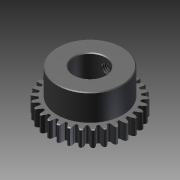
# Autodesk Inventor part: GEAB1.0-30-6-B-12_b
Saved by Autodesk Inventor 2011 SP1 (Build 150282100, 282)
## iProperties
Created: 2016-10-27
Part Number: GEAB1.0-30-6-B-12_b
Catalog Web Link: www.cadenas.de
Description: GEAHB1.0, GEAHBB1.0, GEAHBG1.0, GEAHS1.0, GEAB1.0, GEABB1.0, GEABG1.0, GEAS1.0, GEAKB1.0, GEAKBB1.0, GEAKBG1.0, GEAKS1.0_body-Spur Gears - Pressure Angle 20 Degree Module 1.0
Vendor: MISUMI
Document SubType Name: Modeling
Designer: psAdmin
Manufacturer: MISUMI
Mass: 7.21625 g
Surface Area: 36.7251 cm^2
Volume: 7.21625 cm^3
Density: 1 g/cm^3
Category: PARTsolutions
Company: MISUMI
Title: GEAB1.0-30-6-B-12
Author: Cadenas PARTsolutions
Comments: Spur Gears - Pressure Angle 20 Degree Module 1.0
PSOL_IDENT_0: {$CADENAS_DATA\23d-libs\misumi\metric\54_spur_gears\geab10\geab10.prj},462 {VTYP=3D},{NB=GEAB1.0-30-
PSOL_IDENT_1: 6-B-12_b},{LINA=GEAB1.0-30-6-B-12},{NN=GEAHB1.0, GEAHBB1.0, GEAHBG1.0, GEAHS1.0, GEAB1.0, GEABB1.0,
PSOL_IDENT_2: GEABG1.0, GEAS1.0, GEAKB1.0, GEAKBB1.0, GEAKBG1.0, GEAKS1.0_body},{DATE=13.09.2016 11:19:06},{GEOMDA
PSOL_IDENT_3: TE=13.09.2016 06:08:24},{VERSION=},{LINEID=20},{LINESUBID=-1},{WBVAR=SHS,MAT,ST,NT,B,TS,PS,ALT1,ALT2
PSOL_IDENT_4: ,TPC,ALT11,ALT10,BS,ALT4,Z,J,ALT5,Q,R,S,T,ALT9,SRG,ALT6,LFC,LTC,MALT6,ALT7,KFC,KTC,K,ALT3,DIRALT3,QF
PSOL_IDENT_5: C,QTC,MALT3,ALT8,DIRALT8,ZFC,ZTC,U}  {NB=GEAB1.0-30-6-B-12_b},{LINA=GEAB1.0-30-6-B-12},{KT=DUMMY},{P
PSOL_IDENT_6: N=GEAB1.0-30-6-B-12},{SHS=RHT},{TYPE=GEAB},{MAT=S45C},{MATALG= 'S45C','S45C Equivalent','SUS304','SU
PSOL_IDENT_7: S304' },{ST=},{STALG= '','-','BO','Black Oxide','ENP','Electroless Nickel Plating'},{AC=Set Screw(41
PSOL_IDENT_8: 37 Alloy Steel Black Oxide)},{MOD=1.0},{NT=30},{NTALG=12,13,14,15,16,17,18,19,20,21,22,23,24,25,26,2
PSOL_IDENT_9: 7,28,29,30,32,34,35,36,38,40,42,44,45,46,48,50,52,54,55,56,58,60,62,64,65,66,68,70,72,75,80,84,85,90
PSOL_IDENT_10: ,95,96,100,110,120},{B=6},{BALG=6,8,10,12},{TS=B},{TSALG='B','B'},{TSPN=-B},{PS=12},{PSALG='6','6','
PSOL_IDENT_11: 6.35','6.35','7','7','8','8','9','9','10','10','11','11','12','12','13','13','14','14','15','15','16'
PSOL_IDENT_12: ,'16','17','17'},{P=12.00},{DD=30},{D=32},{G=27.5},{H=25},{L=16},{LL1=10},{LL2=4},{M=M4},{ML=6.500},
PSOL_IDENT_13: {ALT1=},{ALT1ALG='', 'w/o Set Screw', 'KC90','with KC90 (Set Screw)','KC120','with KC120 (Set Screw)'
PSOL_IDENT_14: },{ALT1PN=},{KC=0},{ALT2=},{ALT2ALG= '','w/o TPC (Tapped Hole Dimension)','TPC','with TPC (Tapped H
PSOL_IDENT_15: ole Dimension)' },{TPC=N/A},{TPCALG= 'N/A' },{ALT2PN=},{ALT11=},{ALT11ALG= '', 'w/o GBA (Gear bottom
PSOL_IDENT_16: adjustment of phase focus)','GBA','with GBA (Gear bottom adjustment of phase focus)' },{ALT11PN=},{
PSOL_IDENT_17: DEG=0},{ALT10=},{ALT10ALG= '','w/o BS (Boss Cut)','BS','with BS (Boss Cut)' },{BS=0.0},{BSALG=0},{BS
PSOL_IDENT_18: MIN=7},{BSMAX=10},{ALT10PN=},{LL13D=10},{LL23D=12},{LBS=16},{ALT4=},{ALT4ALG= '','N/A' },{ALT41=0},{
PSOL_IDENT_19: ALT42=0},{ALT4PN=},{Z=0},{ZALG=0},{ZPN=},{ZMINL=14},{ZMAXL=23},{ZMINR=14},{ZMAXR=21},{J=0.0},{JALG=0
PSOL_IDENT_20: },{JPN=},{JMIN=2.0},{JMAX=0.0},{ALT5=},{ALT5ALG= '','N/A' },{ALT5PN=},{Q=0},{QALG=0},{QPN=},{QMIN=14
PSOL_IDENT_21: },{QMAX=21},{R=0},{RALG=0},{RPN=},{RMIN=14},{RMAX=21.0},{S=0},{SALG=0},{SPN=},{SMIN=3},{SMAX=10},{T=
PSOL_IDENT_22: 0},{TALG=0},{TPN=},{TMIN=3},{TMAX=0},{ALT9=},{ALT9ALG= '','Not applicable' },{SRG=0.0},{SRGALG=0},{S
PSOL_IDENT_23: RGMIN=3.500},{SRGMINALG=3.500},{SRGMAX=0.000},{SRGMAXALG=0.000},{DD2=0.0},{MM=0.00},{NN=0.00},{DD2AL
PSOL_IDENT_24: G=0.000},{MMALG=0.000},{NNALG=0.000},{ALT9PN=},{ALT6=},{ALT6ALG= '','N/A' },{ALT6PN=},{LFC=0},{LFCAL
PSOL_IDENT_25: G=0},{LTC=0},{LTCALG=0},{LPCDMIN=20},{LPCDMAX=20},{MALT6=N/A},{MALT6ALG= 'N/A' },{C=0.0},{ALT7=},{AL
PSOL_IDENT_26: T7ALG= '','Not applicable' },{ALT7PN=},{KFC=0},{KFCALG=[0]},{KTC=0},{KTCALG=[0]},{KPCDMIN1=19},{KPCD
PSOL_IDENT_27: MAX1=18},{KPCDMIN2=32},{KPCDMAX2=20},{KPCD=0},{K=0.0},{KALG=[0]},{KALT7L=6},{SCREW=4},{SCREWL=6},{AL
PSOL_IDENT_28: T3=},{ALT3ALG= '','Not applicable' },{DIRALT3=},{DIRALT3ALG= '','N/A' },{ALT3PN=},{QFC=0},{QFCALG=[0
PSOL_IDENT_29: ]},{QTC=0},{QTCALG=[0]},{QPCDMIN1=19},{QPCDMAX1=18},{QPCDMIN2=32},{QPCDMAX2=20},{CIFMALT3=3},{QPCD=0
PSOL_IDENT_30: },{MALT3=N/A},{MALT3ALG= 'N/A' },{MALT3L=0},{MS1=3},{PITCH=0},{BB=4},{TT=0},{ALT8=},{ALT8ALG= '','No
PSOL_IDENT_31: t applicable' },{DIRALT8=},{DIRALT8ALG= '','N/A' },{ALT8PN=},{ZFC=0},{ZFCALG=[0]},{ZFCMIN=22},{ZFCMA
PSOL_IDENT_32: X=17},{ZTC=0},{ZTCALG=[0]},{ZPCDMIN1=22},{ZPCDMIN2=36},{ZPCDMAX1=14},{ZPCDMAX2=17},{ZPCD=0},{U=0},{U
PSOL_IDENT_33: ALG=[0]},{UMAX=0},{UMAX1=0},{UMAX2=6},{UMIN=3},{U1=0.0},{U2=0.0},{F=0.0},{PLANE=6},{BL1=0},{BL2=15.5
PSOL_IDENT_34: },{PCD=0},{SHN=0},{SHDEG1=0},{SHDEG2=0},{PZQRDD2=12},{ALT3LBS=15.5},{D1=3},{D2=6},{D3=20},{D4=0.1},{
PSOL_IDENT_35: D5=5},{D6=4.615385},{D7=0.85},{D8=0.5},{D9=0.820909},{S1=15},{S2=0.5},{KR=18.16}
NN: 0.00
NT: 30
NB: GEAB1.0-30-6-B-12_b
NBSYN: $PN._b
LINA: GEAB1.0-30-6-B-12
PN: GEAB1.0-30-6-B-12
SHS: Round Hole+Tap
MAT: S45C Equivalent
ST: -
AC: Set Screw(4137 Alloy Steel Black Oxide)
MOD: 1.0
B: 6
TS: B
PS: 12
DD: 30
D: 32
G: 27.5
H: 25
L: 16
LL1: 10
LL2: 4
M: M4
ALT1: w/o Set Screw
ALT2: w/o TPC (Tapped Hole Dimension)
TPC: N/A
ALT11: w/o GBA (Gear bottom adjustment of phase focus)
ALT10: w/o BS (Boss Cut)
BS: 0.0
ALT4: N/A
Z: 0
J: 0.0
ALT5: N/A
Q: 0
R: 0
S: 0
T: 0
ALT9: Not applicable
SRG: 0.0
DD2: 0.0
MM: 0.00
ALT6: N/A
LFC: 0
LTC: 0
MALT6: N/A
C: 0.0
ALT7: Not applicable
KFC: 0
KTC: 0
K: 0.0
ALT3: Not applicable
DIRALT3: N/A
QFC: 0
QTC: 0
MALT3: N/A
ALT8: Not applicable
DIRALT8: N/A
ZFC: 0
ZTC: 0
U: 0
U1: 0.0
U2: 0.0
F: 0.0
SUPPLIER: MISUMI
ARTICLENO: GEAB1.0-30-6-B-12_b
BOMINFO: GEAB1.0-30-6-B-12
CREATOR: CADENAS GmbH
Autodesk Inventor part; units mm, degrees
sketch "Sketch_2" plane through (0, 0, 0) normal (1, 0, 0) x (0, 1, 0)
  line L0 (0, -500) -> (0, 500)
  line L1 (0, 16) -> (12.2, 16)
  line L2 (12.2, 16) -> (12.5, 15.7)
  line L3 (12.5, 15.7) -> (12.5, 6)
  line L4 (12.5, 6) -> (15.5, 6)
  line L5 (15.5, 6) -> (21, 4.5263)
  line L6 (21, 4.5263) -> (21, 1.4737)
  line L7 (21, 1.4737) -> (15.5, 0)
  line L8 (15.5, 0) -> (0, 0)
  line L9 (0, 0) -> (0, 16)
  constraints: 20 end point
revolve "Revolution1" add sketch "Sketch_2" angle 360 about axis through (0, 0, -500) along (0, 0, -1)
sketch "Sketch_3" plane through (0, 0, 0) normal (0, 0, 1) x (1, 0, 0)
  circle A0 centre (0, 0) radius 64
  arc A1 (-15.8977, -1.2947) -> (-15.9399, -1.3852) centre (-15.8403, -1.3765) ccw
  arc A2 (-15.9399, -1.3852) -> (-15.8796, -1.9592) centre (0, 0) ccw
  arc A3 (-15.8796, -1.9592) -> (-15.8195, -2.039) centre (-15.7803, -1.9469) ccw
  arc A4 (-15.8195, -2.039) -> (-14.8153, -2.3465) centre (-13.8613, 2.5616) ccw
  arc A5 (-14.8153, -2.3465) -> (-14.6215, -2.3608) centre (-14.6587, -1.5407) ccw
  arc A6 (-13.8996, -2.3851) -> (-14.6215, -2.3608) centre (-14.4159, -6.9716) ccw
  arc A7 (-13.4659, -2.7809) -> (-13.8996, -2.3851) centre (-13.9555, -2.882) ccw
  arc A8 (-13.4659, -2.7809) -> (-13.4328, -2.9366) centre (0, 0) ccw
  arc A9 (-13.668, -3.4745) -> (-13.4328, -2.9366) centre (-13.9212, -3.0434) ccw
  arc A10 (-14.3176, -3.7905) -> (-13.668, -3.4745) centre (-16.0052, 0.5054) ccw
  arc A11 (-14.3176, -3.7905) -> (-14.4889, -3.8823) centre (-14.018, -4.5547) ccw
  arc A12 (-14.4889, -3.8823) -> (-15.2812, -4.5717) centre (-11.621, -7.978) ccw
  arc A13 (-15.2812, -4.5717) -> (-15.3036, -4.669) centre (-15.208, -4.6398) ccw
  arc A14 (-15.3036, -4.669) -> (-15.1252, -5.2179) centre (0, 0) ccw
  arc A15 (-15.1252, -5.2179) -> (-15.0499, -5.2835) centre (-15.0307, -5.1853) ccw
  arc A16 (-15.0499, -5.2835) -> (-14.0037, -5.3755) centre (-14.091, -0.3763) ccw
  arc A17 (-14.0037, -5.3755) -> (-13.8112, -5.3492) centre (-14.018, -4.5547) ccw
  arc A18 (-13.0999, -5.2229) -> (-13.8112, -5.3492) centre (-12.6514, -9.8164) ccw
  arc A19 (-12.5934, -5.5198) -> (-13.0999, -5.2229) centre (-13.0514, -5.7205) ccw
  arc A20 (-12.5934, -5.5198) -> (-12.5287, -5.6652) centre (0, 0) ccw
  arc A21 (-12.647, -6.2403) -> (-12.5287, -5.6652) centre (-12.9843, -5.8713) ccw
  arc A22 (-13.2167, -6.6844) -> (-12.647, -6.2403) centre (-15.7605, -2.8333) ccw
  arc A23 (-13.2167, -6.6844) -> (-13.3651, -6.8099) centre (-12.7647, -7.3697) ccw
  arc A24 (-13.3651, -6.8099) -> (-13.9967, -7.6489) centre (-9.7083, -10.2198) ccw
  arc A25 (-13.9967, -7.6489) -> (-13.9984, -7.7488) centre (-13.911, -7.7003) ccw
  arc A26 (-13.9984, -7.7488) -> (-13.7099, -8.2486) centre (0, 0) ccw
  arc A27 (-13.7099, -8.2486) -> (-13.6225, -8.2971) centre (-13.6242, -8.1971) ccw
  arc A28 (-13.6225, -8.2971) -> (-12.5801, -8.1696) centre (-13.7048, -3.2977) ccw
  arc A29 (-12.5801, -8.1696) -> (-12.3972, -8.1038) centre (-12.7647, -7.3697) ccw
  arc A30 (-11.7278, -7.8324) -> (-12.3972, -8.1038) centre (-10.334, -12.2323) ccw
  arc A31 (-11.1706, -8.0175) -> (-11.7278, -7.8324) centre (-11.5768, -8.3091) ccw
  arc A32 (-11.1706, -8.0175) -> (-11.077, -8.1463) centre (0, 0) ccw
  arc A33 (-11.0731, -8.7334) -> (-11.077, -8.1463) centre (-11.4798, -8.4425) ccw
  arc A34 (-11.5381, -9.2863) -> (-11.0731, -8.7334) centre (-14.827, -6.0482) ccw
  arc A35 (-11.5381, -9.2863) -> (-11.6572, -9.4398) centre (-10.9535, -9.8626) ccw
  arc A36 (-11.6572, -9.4398) -> (-12.1006, -10.3919) centre (-7.3714, -12.015) ccw
  arc A37 (-12.1006, -10.3919) -> (-12.0815, -10.4899) centre (-12.006, -10.4243) ccw
  arc A38 (-12.0815, -10.4899) -> (-11.6953, -10.9188) centre (0, 0) ccw
  arc A39 (-11.6953, -10.9188) -> (-11.5998, -10.948) centre (-11.6222, -10.8506) ccw
  arc A40 (-11.5998, -10.948) -> (-10.6066, -10.6066) centre (-12.7197, -6.0751) ccw
  arc A41 (-10.6066, -10.6066) -> (-10.4415, -10.5042) centre (-10.9535, -9.8626) ccw
  arc A42 (-9.843, -10.0996) -> (-10.4415, -10.5042) centre (-7.5649, -14.1136) ccw
  arc A43 (-9.2595, -10.1648) -> (-9.843, -10.0996) centre (-9.5963, -10.5344) ccw
  arc A44 (-9.2595, -10.1648) -> (-9.1412, -10.2713) centre (0, 0) ccw
  arc A45 (-9.0154, -10.8448) -> (-9.1412, -10.2713) centre (-9.4737, -10.6448) ccw
  arc A46 (-9.3552, -11.4822) -> (-9.0154, -10.8448) centre (-13.2455, -8.9988) ccw
  arc A47 (-9.3552, -11.4822) -> (-9.4398, -11.6572) centre (-8.6636, -11.9245) ccw
  arc A48 (-9.4398, -11.6572) -> (-9.6755, -12.6806) centre (-4.7122, -13.285) ccw
  arc A49 (-9.6755, -12.6806) -> (-9.6365, -12.7725) centre (-9.5763, -12.6927) ccw
  arc A50 (-9.6365, -12.7725) -> (-9.1696, -13.1118) centre (0, 0) ccw
  arc A51 (-9.1696, -13.1118) -> (-9.0701, -13.1205) centre (-9.1122, -13.0298) ccw
  arc A52 (-9.0701, -13.1205) -> (-8.1696, -12.5801) centre (-11.1787, -8.5869) ccw
  arc A53 (-8.1696, -12.5801) -> (-8.0293, -12.4456) centre (-8.6636, -11.9245) ccw
  arc A54 (-7.5281, -11.9254) -> (-8.0293, -12.4456) centre (-4.4652, -15.378) ccw
  arc A55 (-6.9438, -11.8679) -> (-7.5281, -11.9254) centre (-7.1963, -12.2994) ccw
  arc A56 (-6.9438, -11.8679) -> (-6.806, -11.9474) centre (0, 0) ccw
  arc A57 (-6.5636, -12.4822) -> (-6.806, -11.9474) centre (-7.0534, -12.3819) ccw
  arc A58 (-6.7635, -13.1764) -> (-6.5636, -12.4822) centre (-11.0851, -11.556) ccw
  arc A59 (-6.7635, -13.1764) -> (-6.8099, -13.3651) centre (-5.9951, -13.4651) ccw
  arc A60 (-6.8099, -13.3651) -> (-6.8277, -14.4152) centre (-1.8471, -13.9744) ccw
  arc A61 (-6.8277, -14.4152) -> (-6.7704, -14.497) centre (-6.7281, -14.4064) ccw
  arc A62 (-6.7704, -14.497) -> (-6.2431, -14.7317) centre (0, 0) ccw
  arc A63 (-6.2431, -14.7317) -> (-6.144, -14.7196) centre (-6.2041, -14.6397) ccw
  arc A64 (-6.144, -14.7196) -> (-5.3755, -14.0037) centre (-9.1491, -10.7234) ccw
  arc A65 (-5.3755, -14.0037) -> (-5.2663, -13.843) centre (-5.9951, -13.4651) ccw
  arc A66 (-4.8842, -13.23) -> (-5.2663, -13.843) centre (-1.1704, -15.9703) ccw
  arc A67 (-4.3246, -13.0522) -> (-4.8842, -13.23) centre (-4.4819, -13.5268) ccw
  arc A68 (-4.3246, -13.0522) -> (-4.1732, -13.1014) centre (0, 0) ccw
  arc A69 (-3.825, -13.5741) -> (-4.1732, -13.1014) centre (-4.325, -13.5778) ccw
  arc A70 (-3.8762, -14.2947) -> (-3.825, -13.5741) centre (-8.4402, -13.6082) ccw
  arc A71 (-3.8762, -14.2947) -> (-3.8823, -14.4889) centre (-3.0645, -14.4173) ccw
  arc A72 (-3.8823, -14.4889) -> (-3.6814, -15.5197) centre (1.0987, -14.0531) ccw
  arc A73 (-3.6814, -15.5197) -> (-3.6083, -15.5878) centre (-3.5858, -15.4904) ccw
  arc A74 (-3.6083, -15.5878) -> (-3.0438, -15.7078) centre (0, 0) ccw
  arc A75 (-3.0438, -15.7078) -> (-2.9493, -15.6753) centre (-3.0247, -15.6096) ccw
  arc A76 (-2.9493, -15.6753) -> (-2.3465, -14.8153) centre (-6.7196, -12.3913) ccw
  arc A77 (-2.3465, -14.8153) -> (-2.2731, -14.6354) centre (-3.0645, -14.4173) ccw
  arc A78 (-2.0268, -13.9563) -> (-2.2731, -14.6354) centre (2.1756, -15.8647) ccw
  arc A79 (-1.5164, -13.6661) -> (-2.0268, -13.9563) centre (-1.5715, -14.1631) ccw
  arc A80 (-1.5164, -13.6661) -> (-1.3581, -13.6828) centre (0, 0) ccw
  arc A81 (-0.9192, -14.0728) -> (-1.3581, -13.6828) centre (-1.4075, -14.1803) ccw
  arc A82 (-0.8195, -14.7882) -> (-0.9192, -14.0728) centre (-5.4265, -15.0656) ccw
  arc A83 (-0.8195, -14.7882) -> (-0.785, -14.9794) centre (0, -14.7394) ccw
  arc A84 (-0.785, -14.9794) -> (-0.3742, -15.946) centre (3.9965, -13.5176) ccw
  arc A85 (-0.3742, -15.946) -> (-0.2886, -15.9974) centre (-0.2868, -15.8974) ccw
  arc A86 (-0.2886, -15.9974) -> (0.2886, -15.9974) centre (0, 0) ccw
  arc A87 (0.2886, -15.9974) -> (0.3742, -15.946) centre (0.2868, -15.8974) ccw
  arc A88 (0.3742, -15.946) -> (0.785, -14.9794) centre (-3.9965, -13.5176) ccw
  arc A89 (0.785, -14.9794) -> (0.8195, -14.7882) centre (0, -14.7394) ccw
  arc A90 (0.9192, -14.0728) -> (0.8195, -14.7882) centre (5.4265, -15.0656) ccw
  arc A91 (1.3581, -13.6828) -> (0.9192, -14.0728) centre (1.4075, -14.1803) ccw
  arc A92 (1.3581, -13.6828) -> (1.5164, -13.6661) centre (0, 0) ccw
  arc A93 (2.0268, -13.9563) -> (1.5164, -13.6661) centre (1.5715, -14.1631) ccw
  arc A94 (2.2731, -14.6354) -> (2.0268, -13.9563) centre (-2.1756, -15.8647) ccw
  arc A95 (2.2731, -14.6354) -> (2.3465, -14.8153) centre (3.0645, -14.4173) ccw
  arc A96 (2.3465, -14.8153) -> (2.9493, -15.6753) centre (6.7196, -12.3913) ccw
  arc A97 (2.9493, -15.6753) -> (3.0438, -15.7078) centre (3.0247, -15.6096) ccw
  arc A98 (3.0438, -15.7078) -> (3.6083, -15.5878) centre (0, 0) ccw
  arc A99 (3.6083, -15.5878) -> (3.6814, -15.5197) centre (3.5858, -15.4904) ccw
  arc A100 (3.6814, -15.5197) -> (3.8823, -14.4889) centre (-1.0987, -14.0531) ccw
  arc A101 (3.8823, -14.4889) -> (3.8762, -14.2947) centre (3.0645, -14.4173) ccw
  arc A102 (3.825, -13.5741) -> (3.8762, -14.2947) centre (8.4402, -13.6082) ccw
  arc A103 (4.1732, -13.1014) -> (3.825, -13.5741) centre (4.325, -13.5778) ccw
  arc A104 (4.1732, -13.1014) -> (4.3246, -13.0522) centre (0, 0) ccw
  arc A105 (4.8842, -13.23) -> (4.3246, -13.0522) centre (4.4819, -13.5268) ccw
  arc A106 (5.2663, -13.843) -> (4.8842, -13.23) centre (1.1704, -15.9703) ccw
  arc A107 (5.2663, -13.843) -> (5.3755, -14.0037) centre (5.9951, -13.4651) ccw
  arc A108 (5.3755, -14.0037) -> (6.144, -14.7196) centre (9.1491, -10.7234) ccw
  arc A109 (6.144, -14.7196) -> (6.2431, -14.7317) centre (6.2041, -14.6397) ccw
  arc A110 (6.2431, -14.7317) -> (6.7704, -14.497) centre (0, 0) ccw
  arc A111 (6.7704, -14.497) -> (6.8277, -14.4152) centre (6.7281, -14.4064) ccw
  arc A112 (6.8277, -14.4152) -> (6.8099, -13.3651) centre (1.8471, -13.9744) ccw
  arc A113 (6.8099, -13.3651) -> (6.7635, -13.1764) centre (5.9951, -13.4651) ccw
  arc A114 (6.5636, -12.4822) -> (6.7635, -13.1764) centre (11.0851, -11.556) ccw
  arc A115 (6.806, -11.9474) -> (6.5636, -12.4822) centre (7.0534, -12.3819) ccw
  arc A116 (6.806, -11.9474) -> (6.9438, -11.8679) centre (0, 0) ccw
  arc A117 (7.5281, -11.9254) -> (6.9438, -11.8679) centre (7.1963, -12.2994) ccw
  arc A118 (8.0293, -12.4456) -> (7.5281, -11.9254) centre (4.4652, -15.378) ccw
  arc A119 (8.0293, -12.4456) -> (8.1696, -12.5801) centre (8.6636, -11.9245) ccw
  arc A120 (8.1696, -12.5801) -> (9.0701, -13.1205) centre (11.1787, -8.5869) ccw
  arc A121 (9.0701, -13.1205) -> (9.1696, -13.1118) centre (9.1122, -13.0298) ccw
  arc A122 (9.1696, -13.1118) -> (9.6365, -12.7725) centre (0, 0) ccw
  arc A123 (9.6365, -12.7725) -> (9.6755, -12.6806) centre (9.5763, -12.6927) ccw
  arc A124 (9.6755, -12.6806) -> (9.4398, -11.6572) centre (4.7122, -13.285) ccw
  arc A125 (9.4398, -11.6572) -> (9.3552, -11.4822) centre (8.6636, -11.9245) ccw
  arc A126 (9.0154, -10.8448) -> (9.3552, -11.4822) centre (13.2455, -8.9988) ccw
  arc A127 (9.1412, -10.2713) -> (9.0154, -10.8448) centre (9.4737, -10.6448) ccw
  arc A128 (9.1412, -10.2713) -> (9.2595, -10.1648) centre (0, 0) ccw
  arc A129 (9.843, -10.0996) -> (9.2595, -10.1648) centre (9.5963, -10.5344) ccw
  arc A130 (10.4415, -10.5042) -> (9.843, -10.0996) centre (7.5649, -14.1136) ccw
  arc A131 (10.4415, -10.5042) -> (10.6066, -10.6066) centre (10.9535, -9.8626) ccw
  arc A132 (10.6066, -10.6066) -> (11.5998, -10.948) centre (12.7197, -6.0751) ccw
  arc A133 (11.5998, -10.948) -> (11.6953, -10.9188) centre (11.6222, -10.8506) ccw
  arc A134 (11.6953, -10.9188) -> (12.0815, -10.4899) centre (0, 0) ccw
  arc A135 (12.0815, -10.4899) -> (12.1006, -10.3919) centre (12.006, -10.4243) ccw
  arc A136 (12.1006, -10.3919) -> (11.6572, -9.4398) centre (7.3714, -12.015) ccw
  arc A137 (11.6572, -9.4398) -> (11.5381, -9.2863) centre (10.9535, -9.8626) ccw
  arc A138 (11.0731, -8.7334) -> (11.5381, -9.2863) centre (14.827, -6.0482) ccw
  arc A139 (11.077, -8.1463) -> (11.0731, -8.7334) centre (11.4798, -8.4425) ccw
  arc A140 (11.077, -8.1463) -> (11.1706, -8.0175) centre (0, 0) ccw
  arc A141 (11.7278, -7.8324) -> (11.1706, -8.0175) centre (11.5768, -8.3091) ccw
  arc A142 (12.3972, -8.1038) -> (11.7278, -7.8324) centre (10.334, -12.2323) ccw
  arc A143 (12.3972, -8.1038) -> (12.5801, -8.1696) centre (12.7647, -7.3697) ccw
  arc A144 (12.5801, -8.1696) -> (13.6225, -8.2971) centre (13.7048, -3.2977) ccw
  arc A145 (13.6225, -8.2971) -> (13.7099, -8.2486) centre (13.6242, -8.1971) ccw
  arc A146 (13.7099, -8.2486) -> (13.9984, -7.7488) centre (0, 0) ccw
  arc A147 (13.9984, -7.7488) -> (13.9967, -7.6489) centre (13.911, -7.7003) ccw
  arc A148 (13.9967, -7.6489) -> (13.3651, -6.8099) centre (9.7083, -10.2198) ccw
  arc A149 (13.3651, -6.8099) -> (13.2167, -6.6844) centre (12.7647, -7.3697) ccw
  arc A150 (12.647, -6.2403) -> (13.2167, -6.6844) centre (15.7605, -2.8333) ccw
  arc A151 (12.5287, -5.6652) -> (12.647, -6.2403) centre (12.9843, -5.8713) ccw
  arc A152 (12.5287, -5.6652) -> (12.5934, -5.5198) centre (0, 0) ccw
  arc A153 (13.0999, -5.2229) -> (12.5934, -5.5198) centre (13.0514, -5.7205) ccw
  arc A154 (13.8112, -5.3492) -> (13.0999, -5.2229) centre (12.6514, -9.8164) ccw
  arc A155 (13.8112, -5.3492) -> (14.0037, -5.3755) centre (14.018, -4.5547) ccw
  arc A156 (14.0037, -5.3755) -> (15.0499, -5.2835) centre (14.091, -0.3763) ccw
  arc A157 (15.0499, -5.2835) -> (15.1252, -5.2179) centre (15.0307, -5.1853) ccw
  arc A158 (15.1252, -5.2179) -> (15.3036, -4.669) centre (0, 0) ccw
  arc A159 (15.3036, -4.669) -> (15.2812, -4.5717) centre (15.208, -4.6398) ccw
  arc A160 (15.2812, -4.5717) -> (14.4889, -3.8823) centre (11.621, -7.978) ccw
  arc A161 (14.4889, -3.8823) -> (14.3176, -3.7905) centre (14.018, -4.5547) ccw
  arc A162 (13.668, -3.4745) -> (14.3176, -3.7905) centre (16.0052, 0.5054) ccw
  arc A163 (13.4328, -2.9366) -> (13.668, -3.4745) centre (13.9212, -3.0434) ccw
  arc A164 (13.4328, -2.9366) -> (13.4659, -2.7809) centre (0, 0) ccw
  arc A165 (13.8996, -2.3851) -> (13.4659, -2.7809) centre (13.9555, -2.882) ccw
  arc A166 (14.6215, -2.3608) -> (13.8996, -2.3851) centre (14.4159, -6.9716) ccw
  arc A167 (14.6215, -2.3608) -> (14.8153, -2.3465) centre (14.6587, -1.5407) ccw
  arc A168 (14.8153, -2.3465) -> (15.8195, -2.039) centre (13.8613, 2.5616) ccw
  arc A169 (15.8195, -2.039) -> (15.8796, -1.9592) centre (15.7803, -1.9469) ccw
  arc A170 (15.8796, -1.9592) -> (15.9399, -1.3852) centre (0, 0) ccw
  arc A171 (15.9399, -1.3852) -> (15.8977, -1.2947) centre (15.8403, -1.3765) ccw
  arc A172 (15.8977, -1.2947) -> (14.9794, -0.785) centre (13.0258, -5.3876) ccw
  arc A173 (14.9794, -0.785) -> (14.7929, -0.7308) centre (14.6587, -1.5407) ccw
  arc A174 (14.0917, -0.5569) -> (14.7929, -0.7308) centre (15.5503, 3.822) ccw
  arc A175 (13.7498, -0.0796) -> (14.0917, -0.5569) centre (14.2498, -0.0825) ccw
  arc A176 (13.7498, -0.0796) -> (13.7498, 0.0796) centre (0, 0) ccw
  arc A177 (14.0917, 0.5569) -> (13.7498, 0.0796) centre (14.2498, 0.0825) ccw
  arc A178 (14.7929, 0.7308) -> (14.0917, 0.5569) centre (15.5503, -3.822) ccw
  arc A179 (14.7929, 0.7308) -> (14.9794, 0.785) centre (14.6587, 1.5407) ccw
  arc A180 (14.9794, 0.785) -> (15.8977, 1.2947) centre (13.0258, 5.3876) ccw
  arc A181 (15.8977, 1.2947) -> (15.9399, 1.3852) centre (15.8403, 1.3765) ccw
  arc A182 (15.9399, 1.3852) -> (15.8796, 1.9592) centre (0, 0) ccw
  arc A183 (15.8796, 1.9592) -> (15.8195, 2.039) centre (15.7803, 1.9469) ccw
  arc A184 (15.8195, 2.039) -> (14.8153, 2.3465) centre (13.8613, -2.5616) ccw
  arc A185 (14.8153, 2.3465) -> (14.6215, 2.3608) centre (14.6587, 1.5407) ccw
  arc A186 (13.8996, 2.3851) -> (14.6215, 2.3608) centre (14.4159, 6.9716) ccw
  arc A187 (13.4659, 2.7809) -> (13.8996, 2.3851) centre (13.9555, 2.882) ccw
  arc A188 (13.4659, 2.7809) -> (13.4328, 2.9366) centre (0, 0) ccw
  arc A189 (13.668, 3.4745) -> (13.4328, 2.9366) centre (13.9212, 3.0434) ccw
  arc A190 (14.3176, 3.7905) -> (13.668, 3.4745) centre (16.0052, -0.5054) ccw
  arc A191 (14.3176, 3.7905) -> (14.4889, 3.8823) centre (14.018, 4.5547) ccw
  arc A192 (14.4889, 3.8823) -> (15.2812, 4.5717) centre (11.621, 7.978) ccw
  arc A193 (15.2812, 4.5717) -> (15.3036, 4.669) centre (15.208, 4.6398) ccw
  arc A194 (15.3036, 4.669) -> (15.1252, 5.2179) centre (0, 0) ccw
  arc A195 (15.1252, 5.2179) -> (15.0499, 5.2835) centre (15.0307, 5.1853) ccw
  arc A196 (15.0499, 5.2835) -> (14.0037, 5.3755) centre (14.091, 0.3763) ccw
  arc A197 (14.0037, 5.3755) -> (13.8112, 5.3492) centre (14.018, 4.5547) ccw
  arc A198 (13.0999, 5.2229) -> (13.8112, 5.3492) centre (12.6514, 9.8164) ccw
  arc A199 (12.5934, 5.5198) -> (13.0999, 5.2229) centre (13.0514, 5.7205) ccw
  arc A200 (12.5934, 5.5198) -> (12.5287, 5.6652) centre (0, 0) ccw
  arc A201 (12.647, 6.2403) -> (12.5287, 5.6652) centre (12.9843, 5.8713) ccw
  arc A202 (13.2167, 6.6844) -> (12.647, 6.2403) centre (15.7605, 2.8333) ccw
  arc A203 (13.2167, 6.6844) -> (13.3651, 6.8099) centre (12.7647, 7.3697) ccw
  arc A204 (13.3651, 6.8099) -> (13.9967, 7.6489) centre (9.7083, 10.2198) ccw
  arc A205 (13.9967, 7.6489) -> (13.9984, 7.7488) centre (13.911, 7.7003) ccw
  arc A206 (13.9984, 7.7488) -> (13.7099, 8.2486) centre (0, 0) ccw
  arc A207 (13.7099, 8.2486) -> (13.6225, 8.2971) centre (13.6242, 8.1971) ccw
  arc A208 (13.6225, 8.2971) -> (12.5801, 8.1696) centre (13.7048, 3.2977) ccw
  arc A209 (12.5801, 8.1696) -> (12.3972, 8.1038) centre (12.7647, 7.3697) ccw
  arc A210 (11.7278, 7.8324) -> (12.3972, 8.1038) centre (10.334, 12.2323) ccw
  arc A211 (11.1706, 8.0175) -> (11.7278, 7.8324) centre (11.5768, 8.3091) ccw
  arc A212 (11.1706, 8.0175) -> (11.077, 8.1463) centre (0, 0) ccw
  arc A213 (11.0731, 8.7334) -> (11.077, 8.1463) centre (11.4798, 8.4425) ccw
  arc A214 (11.5381, 9.2863) -> (11.0731, 8.7334) centre (14.827, 6.0482) ccw
  arc A215 (11.5381, 9.2863) -> (11.6572, 9.4398) centre (10.9535, 9.8626) ccw
  arc A216 (11.6572, 9.4398) -> (12.1006, 10.3919) centre (7.3714, 12.015) ccw
  arc A217 (12.1006, 10.3919) -> (12.0815, 10.4899) centre (12.006, 10.4243) ccw
  arc A218 (12.0815, 10.4899) -> (11.6953, 10.9188) centre (0, 0) ccw
  arc A219 (11.6953, 10.9188) -> (11.5998, 10.948) centre (11.6222, 10.8506) ccw
  arc A220 (11.5998, 10.948) -> (10.6066, 10.6066) centre (12.7197, 6.0751) ccw
  arc A221 (10.6066, 10.6066) -> (10.4415, 10.5042) centre (10.9535, 9.8626) ccw
  arc A222 (9.843, 10.0996) -> (10.4415, 10.5042) centre (7.5649, 14.1136) ccw
  arc A223 (9.2595, 10.1648) -> (9.843, 10.0996) centre (9.5963, 10.5344) ccw
  arc A224 (9.2595, 10.1648) -> (9.1412, 10.2713) centre (0, 0) ccw
  arc A225 (9.0154, 10.8448) -> (9.1412, 10.2713) centre (9.4737, 10.6448) ccw
  arc A226 (9.3552, 11.4822) -> (9.0154, 10.8448) centre (13.2455, 8.9988) ccw
  arc A227 (9.3552, 11.4822) -> (9.4398, 11.6572) centre (8.6636, 11.9245) ccw
  arc A228 (9.4398, 11.6572) -> (9.6755, 12.6806) centre (4.7122, 13.285) ccw
  arc A229 (9.6755, 12.6806) -> (9.6365, 12.7725) centre (9.5763, 12.6927) ccw
  arc A230 (9.6365, 12.7725) -> (9.1696, 13.1118) centre (0, 0) ccw
  arc A231 (9.1696, 13.1118) -> (9.0701, 13.1205) centre (9.1122, 13.0298) ccw
  arc A232 (9.0701, 13.1205) -> (8.1696, 12.5801) centre (11.1787, 8.5869) ccw
  arc A233 (8.1696, 12.5801) -> (8.0293, 12.4456) centre (8.6636, 11.9245) ccw
  arc A234 (7.5281, 11.9254) -> (8.0293, 12.4456) centre (4.4652, 15.378) ccw
  arc A235 (6.9438, 11.8679) -> (7.5281, 11.9254) centre (7.1963, 12.2994) ccw
  arc A236 (6.9438, 11.8679) -> (6.806, 11.9474) centre (0, 0) ccw
  arc A237 (6.5636, 12.4822) -> (6.806, 11.9474) centre (7.0534, 12.3819) ccw
  arc A238 (6.7635, 13.1764) -> (6.5636, 12.4822) centre (11.0851, 11.556) ccw
  arc A239 (6.7635, 13.1764) -> (6.8099, 13.3651) centre (5.9951, 13.4651) ccw
  arc A240 (6.8099, 13.3651) -> (6.8277, 14.4152) centre (1.8471, 13.9744) ccw
  arc A241 (6.8277, 14.4152) -> (6.7704, 14.497) centre (6.7281, 14.4064) ccw
  arc A242 (6.7704, 14.497) -> (6.2431, 14.7317) centre (0, 0) ccw
  arc A243 (6.2431, 14.7317) -> (6.144, 14.7196) centre (6.2041, 14.6397) ccw
  arc A244 (6.144, 14.7196) -> (5.3755, 14.0037) centre (9.1491, 10.7234) ccw
  arc A245 (5.3755, 14.0037) -> (5.2663, 13.843) centre (5.9951, 13.4651) ccw
  arc A246 (4.8842, 13.23) -> (5.2663, 13.843) centre (1.1704, 15.9703) ccw
  arc A247 (4.3246, 13.0522) -> (4.8842, 13.23) centre (4.4819, 13.5268) ccw
  arc A248 (4.3246, 13.0522) -> (4.1732, 13.1014) centre (0, 0) ccw
  arc A249 (3.825, 13.5741) -> (4.1732, 13.1014) centre (4.325, 13.5778) ccw
  arc A250 (3.8762, 14.2947) -> (3.825, 13.5741) centre (8.4402, 13.6082) ccw
  arc A251 (3.8762, 14.2947) -> (3.8823, 14.4889) centre (3.0645, 14.4173) ccw
  arc A252 (3.8823, 14.4889) -> (3.6814, 15.5197) centre (-1.0987, 14.0531) ccw
  arc A253 (3.6814, 15.5197) -> (3.6083, 15.5878) centre (3.5858, 15.4904) ccw
  arc A254 (3.6083, 15.5878) -> (3.0438, 15.7078) centre (0, 0) ccw
  arc A255 (3.0438, 15.7078) -> (2.9493, 15.6753) centre (3.0247, 15.6096) ccw
  arc A256 (2.9493, 15.6753) -> (2.3465, 14.8153) centre (6.7196, 12.3913) ccw
  arc A257 (2.3465, 14.8153) -> (2.2731, 14.6354) centre (3.0645, 14.4173) ccw
  arc A258 (2.0268, 13.9563) -> (2.2731, 14.6354) centre (-2.1756, 15.8647) ccw
  arc A259 (1.5164, 13.6661) -> (2.0268, 13.9563) centre (1.5715, 14.1631) ccw
  arc A260 (1.5164, 13.6661) -> (1.3581, 13.6828) centre (0, 0) ccw
  arc A261 (0.9192, 14.0728) -> (1.3581, 13.6828) centre (1.4075, 14.1803) ccw
  arc A262 (0.8195, 14.7882) -> (0.9192, 14.0728) centre (5.4265, 15.0656) ccw
  arc A263 (0.8195, 14.7882) -> (0.785, 14.9794) centre (0, 14.7394) ccw
  arc A264 (0.785, 14.9794) -> (0.3742, 15.946) centre (-3.9965, 13.5176) ccw
  arc A265 (0.3742, 15.946) -> (0.2886, 15.9974) centre (0.2868, 15.8974) ccw
  arc A266 (0.2886, 15.9974) -> (-0.2886, 15.9974) centre (0, 0) ccw
  arc A267 (-0.2886, 15.9974) -> (-0.3742, 15.946) centre (-0.2868, 15.8974) ccw
  arc A268 (-0.3742, 15.946) -> (-0.785, 14.9794) centre (3.9965, 13.5176) ccw
  arc A269 (-0.785, 14.9794) -> (-0.8195, 14.7882) centre (0, 14.7394) ccw
  arc A270 (-0.9192, 14.0728) -> (-0.8195, 14.7882) centre (-5.4265, 15.0656) ccw
  arc A271 (-1.3581, 13.6828) -> (-0.9192, 14.0728) centre (-1.4075, 14.1803) ccw
  arc A272 (-1.3581, 13.6828) -> (-1.5164, 13.6661) centre (0, 0) ccw
  arc A273 (-2.0268, 13.9563) -> (-1.5164, 13.6661) centre (-1.5715, 14.1631) ccw
  arc A274 (-2.2731, 14.6354) -> (-2.0268, 13.9563) centre (2.1756, 15.8647) ccw
  arc A275 (-2.2731, 14.6354) -> (-2.3465, 14.8153) centre (-3.0645, 14.4173) ccw
  arc A276 (-2.3465, 14.8153) -> (-2.9493, 15.6753) centre (-6.7196, 12.3913) ccw
  arc A277 (-2.9493, 15.6753) -> (-3.0438, 15.7078) centre (-3.0247, 15.6096) ccw
  arc A278 (-3.0438, 15.7078) -> (-3.6083, 15.5878) centre (0, 0) ccw
  arc A279 (-3.6083, 15.5878) -> (-3.6814, 15.5197) centre (-3.5858, 15.4904) ccw
  arc A280 (-3.6814, 15.5197) -> (-3.8823, 14.4889) centre (1.0987, 14.0531) ccw
  arc A281 (-3.8823, 14.4889) -> (-3.8762, 14.2947) centre (-3.0645, 14.4173) ccw
  arc A282 (-3.825, 13.5741) -> (-3.8762, 14.2947) centre (-8.4402, 13.6082) ccw
  arc A283 (-4.1732, 13.1014) -> (-3.825, 13.5741) centre (-4.325, 13.5778) ccw
  arc A284 (-4.1732, 13.1014) -> (-4.3246, 13.0522) centre (0, 0) ccw
  arc A285 (-4.8842, 13.23) -> (-4.3246, 13.0522) centre (-4.4819, 13.5268) ccw
  arc A286 (-5.2663, 13.843) -> (-4.8842, 13.23) centre (-1.1704, 15.9703) ccw
  arc A287 (-5.2663, 13.843) -> (-5.3755, 14.0037) centre (-5.9951, 13.4651) ccw
  arc A288 (-5.3755, 14.0037) -> (-6.144, 14.7196) centre (-9.1491, 10.7234) ccw
  arc A289 (-6.144, 14.7196) -> (-6.2431, 14.7317) centre (-6.2041, 14.6397) ccw
  arc A290 (-6.2431, 14.7317) -> (-6.7704, 14.497) centre (0, 0) ccw
  arc A291 (-6.7704, 14.497) -> (-6.8277, 14.4152) centre (-6.7281, 14.4064) ccw
  arc A292 (-6.8277, 14.4152) -> (-6.8099, 13.3651) centre (-1.8471, 13.9744) ccw
  arc A293 (-6.8099, 13.3651) -> (-6.7635, 13.1764) centre (-5.9951, 13.4651) ccw
  arc A294 (-6.5636, 12.4822) -> (-6.7635, 13.1764) centre (-11.0851, 11.556) ccw
  arc A295 (-6.806, 11.9474) -> (-6.5636, 12.4822) centre (-7.0534, 12.3819) ccw
  arc A296 (-6.806, 11.9474) -> (-6.9438, 11.8679) centre (0, 0) ccw
  arc A297 (-7.5281, 11.9254) -> (-6.9438, 11.8679) centre (-7.1963, 12.2994) ccw
  arc A298 (-8.0293, 12.4456) -> (-7.5281, 11.9254) centre (-4.4652, 15.378) ccw
  arc A299 (-8.0293, 12.4456) -> (-8.1696, 12.5801) centre (-8.6636, 11.9245) ccw
  arc A300 (-8.1696, 12.5801) -> (-9.0701, 13.1205) centre (-11.1787, 8.5869) ccw
  arc A301 (-9.0701, 13.1205) -> (-9.1696, 13.1118) centre (-9.1122, 13.0298) ccw
  arc A302 (-9.1696, 13.1118) -> (-9.6365, 12.7725) centre (0, 0) ccw
  arc A303 (-9.6365, 12.7725) -> (-9.6755, 12.6806) centre (-9.5763, 12.6927) ccw
  arc A304 (-9.6755, 12.6806) -> (-9.4398, 11.6572) centre (-4.7122, 13.285) ccw
  arc A305 (-9.4398, 11.6572) -> (-9.3552, 11.4822) centre (-8.6636, 11.9245) ccw
  arc A306 (-9.0154, 10.8448) -> (-9.3552, 11.4822) centre (-13.2455, 8.9988) ccw
  arc A307 (-9.1412, 10.2713) -> (-9.0154, 10.8448) centre (-9.4737, 10.6448) ccw
  arc A308 (-9.1412, 10.2713) -> (-9.2595, 10.1648) centre (0, 0) ccw
  arc A309 (-9.843, 10.0996) -> (-9.2595, 10.1648) centre (-9.5963, 10.5344) ccw
  arc A310 (-10.4415, 10.5042) -> (-9.843, 10.0996) centre (-7.5649, 14.1136) ccw
  arc A311 (-10.4415, 10.5042) -> (-10.6066, 10.6066) centre (-10.9535, 9.8626) ccw
  arc A312 (-10.6066, 10.6066) -> (-11.5998, 10.948) centre (-12.7197, 6.0751) ccw
  arc A313 (-11.5998, 10.948) -> (-11.6953, 10.9188) centre (-11.6222, 10.8506) ccw
  arc A314 (-11.6953, 10.9188) -> (-12.0815, 10.4899) centre (0, 0) ccw
  arc A315 (-12.0815, 10.4899) -> (-12.1006, 10.3919) centre (-12.006, 10.4243) ccw
  arc A316 (-12.1006, 10.3919) -> (-11.6572, 9.4398) centre (-7.3714, 12.015) ccw
  arc A317 (-11.6572, 9.4398) -> (-11.5381, 9.2863) centre (-10.9535, 9.8626) ccw
  arc A318 (-11.0731, 8.7334) -> (-11.5381, 9.2863) centre (-14.827, 6.0482) ccw
  arc A319 (-11.077, 8.1463) -> (-11.0731, 8.7334) centre (-11.4798, 8.4425) ccw
  arc A320 (-11.077, 8.1463) -> (-11.1706, 8.0175) centre (0, 0) ccw
  arc A321 (-11.7278, 7.8324) -> (-11.1706, 8.0175) centre (-11.5768, 8.3091) ccw
  arc A322 (-12.3972, 8.1038) -> (-11.7278, 7.8324) centre (-10.334, 12.2323) ccw
  arc A323 (-12.3972, 8.1038) -> (-12.5801, 8.1696) centre (-12.7647, 7.3697) ccw
  arc A324 (-12.5801, 8.1696) -> (-13.6225, 8.2971) centre (-13.7048, 3.2977) ccw
  arc A325 (-13.6225, 8.2971) -> (-13.7099, 8.2486) centre (-13.6242, 8.1971) ccw
  arc A326 (-13.7099, 8.2486) -> (-13.9984, 7.7488) centre (0, 0) ccw
  arc A327 (-13.9984, 7.7488) -> (-13.9967, 7.6489) centre (-13.911, 7.7003) ccw
  arc A328 (-13.9967, 7.6489) -> (-13.3651, 6.8099) centre (-9.7083, 10.2198) ccw
  arc A329 (-13.3651, 6.8099) -> (-13.2167, 6.6844) centre (-12.7647, 7.3697) ccw
  arc A330 (-12.647, 6.2403) -> (-13.2167, 6.6844) centre (-15.7605, 2.8333) ccw
  arc A331 (-12.5287, 5.6652) -> (-12.647, 6.2403) centre (-12.9843, 5.8713) ccw
  arc A332 (-12.5287, 5.6652) -> (-12.5934, 5.5198) centre (0, 0) ccw
  arc A333 (-13.0999, 5.2229) -> (-12.5934, 5.5198) centre (-13.0514, 5.7205) ccw
  arc A334 (-13.8112, 5.3492) -> (-13.0999, 5.2229) centre (-12.6514, 9.8164) ccw
  arc A335 (-13.8112, 5.3492) -> (-14.0037, 5.3755) centre (-14.018, 4.5547) ccw
  arc A336 (-14.0037, 5.3755) -> (-15.0499, 5.2835) centre (-14.091, 0.3763) ccw
  arc A337 (-15.0499, 5.2835) -> (-15.1252, 5.2179) centre (-15.0307, 5.1853) ccw
  arc A338 (-15.1252, 5.2179) -> (-15.3036, 4.669) centre (0, 0) ccw
  arc A339 (-15.3036, 4.669) -> (-15.2812, 4.5717) centre (-15.208, 4.6398) ccw
  arc A340 (-15.2812, 4.5717) -> (-14.4889, 3.8823) centre (-11.621, 7.978) ccw
  arc A341 (-14.4889, 3.8823) -> (-14.3176, 3.7905) centre (-14.018, 4.5547) ccw
  arc A342 (-13.668, 3.4745) -> (-14.3176, 3.7905) centre (-16.0052, -0.5054) ccw
  arc A343 (-13.4328, 2.9366) -> (-13.668, 3.4745) centre (-13.9212, 3.0434) ccw
  arc A344 (-13.4328, 2.9366) -> (-13.4659, 2.7809) centre (0, 0) ccw
  arc A345 (-13.8996, 2.3851) -> (-13.4659, 2.7809) centre (-13.9555, 2.882) ccw
  arc A346 (-14.6215, 2.3608) -> (-13.8996, 2.3851) centre (-14.4159, 6.9716) ccw
  arc A347 (-14.6215, 2.3608) -> (-14.8153, 2.3465) centre (-14.6587, 1.5407) ccw
  arc A348 (-14.8153, 2.3465) -> (-15.8195, 2.039) centre (-13.8613, -2.5616) ccw
  arc A349 (-15.8195, 2.039) -> (-15.8796, 1.9592) centre (-15.7803, 1.9469) ccw
  arc A350 (-15.8796, 1.9592) -> (-15.9399, 1.3852) centre (0, 0) ccw
  arc A351 (-15.9399, 1.3852) -> (-15.8977, 1.2947) centre (-15.8403, 1.3765) ccw
  arc A352 (-15.8977, 1.2947) -> (-14.9794, 0.785) centre (-13.0258, 5.3876) ccw
  arc A353 (-14.9794, 0.785) -> (-14.7929, 0.7308) centre (-14.6587, 1.5407) ccw
  arc A354 (-14.0917, 0.5569) -> (-14.7929, 0.7308) centre (-15.5503, -3.822) ccw
  arc A355 (-13.7498, 0.0796) -> (-14.0917, 0.5569) centre (-14.2498, 0.0825) ccw
  arc A356 (-13.7498, 0.0796) -> (-13.7498, -0.0796) centre (0, 0) ccw
  arc A357 (-14.0917, -0.5569) -> (-13.7498, -0.0796) centre (-14.2498, -0.0825) ccw
  arc A358 (-14.7929, -0.7308) -> (-14.0917, -0.5569) centre (-15.5503, 3.822) ccw
  arc A359 (-14.7929, -0.7308) -> (-14.9794, -0.785) centre (-14.6587, -1.5407) ccw
  arc A360 (-14.9794, -0.785) -> (-15.8977, -1.2947) centre (-13.0258, -5.3876) ccw
  constraints: 720 point on circle, 361 centre point
extrude "Extrusion1" cut sketch "Sketch_3" along normal blind 6
sketch "Sketch3" plane through (0, 0, 0) normal (0, 0, -1) x (-0.9945, -0.1045, 0)
  point P0 (0, 0)
hole "Hole1" at (0, 0, 0) direction (0, 0, 1) diameter 12 depth 16
sketch "_____7" plane through (0, 0, 0) normal (1, 0, 0) x (0, 0, -1)
  line L0 (500, 0) -> (-500, 0)
  line L1 (-0.3, 6) -> (0, 6)
  line L2 (0, 6) -> (0, 6.3)
  line L3 (0, 6.3) -> (-0.3, 6)
  constraints: 8 end point
revolve "Revolution2" cut sketch "_____7" angle 360 about axis through (0, 0, -500) along (0, 0, -1)
sketch "_____17" plane through (0, 0, 0) normal (1, 0, 0) x (0, 0, -1)
  line L0 (500, 0) -> (-500, 0)
  line L1 (-16, 6) -> (-15.7, 6)
  line L2 (-15.7, 6) -> (-16, 6.3)
  line L3 (-16, 6.3) -> (-16, 6)
  constraints: 8 end point
revolve "Revolution3" cut sketch "_____17" angle 360 about axis through (0, 0, -500) along (0, 0, -1)
sketch "Sketch_4" plane through (0, 0, 12) normal (0, 0, 1) x (1, 0, 0)
  line L0 (0, 12.5) -> (0, 0)
  line L1 (0, 0) -> (-1.621, 0)
  line L2 (-1.621, 0) -> (-1.621, 12.121)
  line L3 (-1.621, 12.121) -> (-2, 12.5)
  line L4 (-2, 12.5) -> (0, 12.5)
  line L5 (0, 12.5) -> (0, 0)
  constraints: 12 end point
revolve "Revolution4" cut sketch "Sketch_4" angle 360 about axis through (0, 12.5, 12) along (0, 1, 0)
thread "Thread1" size "M4x0.7" class "6H" standard "ISO Metric profile" length 6.121
ref_plane "b_XY" through (0, 0, 0) normal (0, 0, 1) x (1, 0, 0)
ref_plane "b_YZ" through (0, 0, 0) normal (1, 0, 0) x (0, 1, 0)
ref_plane "b_ZX" through (0, 0, 0) normal (0, 1, 0) x (0, 0, 1)
ref_plane "screw_XY" through (0, 6, 12) normal (0, 1, 0) x (1, 0, 0)
ref_plane "screw_YZ" through (0, 6, 12) normal (1, 0, 0) x (0, 0, -1)
ref_plane "screw_ZX" through (0, 6, 12) normal (0, 0, -1) x (0, 1, 0)
ref_plane "turn_around_XY" through (0, 0, 0) normal (-1, 0, 0) x (0, 0, -1)
ref_plane "turn_around_YZ" through (0, 0, 0) normal (0, 0, -1) x (0, -1, 0)
ref_plane "turn_around_ZX" through (0, 0, 0) normal (0, -1, 0) x (-1, 0, 0)
body "Solid1"
